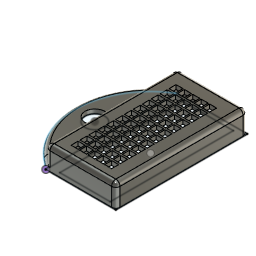
toe-chassis_v1 (Autodesk Fusion 360 design; units mm, degrees)
Autodesk Fusion 360 part; units mm, degrees
sketch "Sketch1" plane through (0, 0, 0) normal (0, 0, 1) x (1, 0, 0)
  line L0 (0, 0) -> (25, 0)
  line L1 (25, 0) -> (25, 47)
  line L2 (25, 47) -> (0, 47)
  line L3 (0, 47) -> (0, 0)
  line L4 (3.5, 1.5) -> (21.5, 1.5)
  line L5 (21.5, 1.5) -> (21.5, 45.5)
  line L6 (21.5, 45.5) -> (3.5, 45.5)
  line L7 (3.5, 45.5) -> (3.5, 1.5)
  line L8 (0, 47) -> (-0.5238, 46.6753)
  line L9 (-3.5824, 2.9853) -> (0, 0)
  arc A0 (-0.5238, 46.6753) -> (-3.5824, 2.9853) centre (13.7026, 23.7273) ccw
  circle A1 centre (-6, 23.5) radius 3.5
  dimension "d1" = 25
  dimension "d2" = 47
  dimension "d3" = 18
  dimension "d4" = 44
  dimension "d5" = 1.5
  dimension "d6" = 3.5
  dimension "d7" = 27
  dimension "d19" = 7
  dimension "d20" = 6
  dimension "d21" = 23.5
  constraint horizontal L0
  constraint vertical L1
  constraint horizontal L2
  constraint vertical L3
  constraint coincident L0.start L3.end
  constraint horizontal L4
  constraint vertical L5
  constraint horizontal L6
  constraint vertical L7
  constraint tangent L9 A0
  constraint tangent L8 A0
  measures "d1" distance of L1.end L2.end
  measures "d2" distance of L0.end L1.end
  measures "d3" distance of L5.end L6.end
  measures "d4" distance of L4.end L5.end
  measures "d5" distance of L2 L6
  measures "d6" distance of L1 L5
  measures "d7" radius of A0
  measures "d19" diameter of A1
  measures "d20" distance of L3 A1.centre
  measures "d21" distance of L2 A1.centre
extrude "Extrude1" add sketch "Sketch1" along normal blind 1.5 contours L0 L1 L2 L3 | L3 L8 L9 A0 | L4 L5 L6 L7 | A1
extrude "Extrude2" add sketch "Sketch1" along normal blind 8 contours L0 L1 L2 L3 | L4 L5 L6 L7
extrude "Extrude3" cut sketch "Sketch1" along normal blind 6.5 contours L4 L5 L6 L7
sketch "Sketch3" plane through (0, 47, 0) normal (0, 1, 0) x (-1, 0, 0)
  line L0 (-25, 0) -> (0, 0)
  line L1 (0, 0) -> (0, 1.5)
  line L2 (0, 1.5) -> (0, 8)
  line L3 (0, 8) -> (-25, 8)
  line L4 (-25, 8) -> (-25, 0)
  line L5 (-17, 0) -> (-8, 0)
  line L6 (-8, 0) -> (-8, 5)
  line L7 (-8, 5) -> (-17, 5)
  line L8 (-17, 5) -> (-17, 0)
  dimension "d14" = 9
  dimension "d15" = 5
  dimension "d16" = 8
  constraint horizontal L5
  constraint vertical L6
  constraint horizontal L7
  constraint vertical L8
  constraint coincident L0 L5.start
  measures "d14" distance of L6.end L7.end
  measures "d15" distance of L5.end L6.end
  measures "d16" distance of L4 L8
extrude "Extrude4" cut sketch "Sketch3" against normal blind 6 contours L0 L5 L6 L7 L8
extrude "Extrude5" cut sketch "Sketch1" along normal blind 8 contours A1
fillet "Fillet1" radius 1.5 8 edges at (0, 47, 4.75) (12.5, 47, 8) (25, 47, 4) (0, 23.5, 8) (25, 23.5, 8) (25, 0, 4) (12.5, 0, 8) (0, 0, 4.75)
fillet "Fillet2" radius 1.5 3 edges at (-0.2619, 46.8376, 1.5) (-13.2315, 25.6129, 1.5) (-1.7912, 1.4927, 1.5)
sketch "Sketch4" plane through (0, 0, 8) normal (0, 0, 1) x (-1, 0, 0)
  line L0 (-1.5, -1.5) -> (-23.5, -1.5)
  line L1 (-23.5, -1.5) -> (-23.5, -45.5)
  line L2 (-23.5, -45.5) -> (-1.5, -45.5)
  line L3 (-1.5, -45.5) -> (-1.5, -1.5)
  line L4 (-19.5, -41.5) -> (-17, -41.5)
  line L5 (-17, -41.5) -> (-17, -39)
  line L6 (-17, -39) -> (-19.5, -39)
  line L7 (-19.5, -39) -> (-19.5, -41.5)
  line L8 (-14, -39) -> (-16.5, -39)
  line L9 (-14, -41.5) -> (-14, -39)
  line L10 (-16.5, -41.5) -> (-14, -41.5)
  line L11 (-16.5, -39) -> (-16.5, -41.5)
  line L12 (-11, -39) -> (-13.5, -39)
  line L13 (-11, -41.5) -> (-11, -39)
  line L14 (-13.5, -41.5) -> (-11, -41.5)
  line L15 (-13.5, -39) -> (-13.5, -41.5)
  line L16 (-8, -39) -> (-10.5, -39)
  line L17 (-8, -41.5) -> (-8, -39)
  line L18 (-10.5, -41.5) -> (-8, -41.5)
  line L19 (-10.5, -39) -> (-10.5, -41.5)
  line L20 (-5, -39) -> (-7.5, -39)
  line L21 (-5, -41.5) -> (-5, -39)
  line L22 (-7.5, -41.5) -> (-5, -41.5)
  line L23 (-7.5, -39) -> (-7.5, -41.5)
  line L24 (-17, -35.8182) -> (-19.5, -35.8182)
  line L25 (-17, -38.3182) -> (-17, -35.8182)
  line L26 (-19.5, -38.3182) -> (-17, -38.3182)
  line L27 (-19.5, -35.8182) -> (-19.5, -38.3182)
  line L28 (-14, -35.8182) -> (-16.5, -35.8182)
  line L29 (-14, -38.3182) -> (-14, -35.8182)
  line L30 (-16.5, -38.3182) -> (-14, -38.3182)
  line L31 (-16.5, -35.8182) -> (-16.5, -38.3182)
  line L32 (-11, -35.8182) -> (-13.5, -35.8182)
  line L33 (-11, -38.3182) -> (-11, -35.8182)
  line L34 (-13.5, -38.3182) -> (-11, -38.3182)
  line L35 (-13.5, -35.8182) -> (-13.5, -38.3182)
  line L36 (-8, -35.8182) -> (-10.5, -35.8182)
  line L37 (-8, -38.3182) -> (-8, -35.8182)
  line L38 (-10.5, -38.3182) -> (-8, -38.3182)
  line L39 (-10.5, -35.8182) -> (-10.5, -38.3182)
  line L40 (-5, -35.8182) -> (-7.5, -35.8182)
  line L41 (-5, -38.3182) -> (-5, -35.8182)
  line L42 (-7.5, -38.3182) -> (-5, -38.3182)
  line L43 (-7.5, -35.8182) -> (-7.5, -38.3182)
  line L44 (-17, -32.6364) -> (-19.5, -32.6364)
  line L45 (-17, -35.1364) -> (-17, -32.6364)
  line L46 (-19.5, -35.1364) -> (-17, -35.1364)
  line L47 (-19.5, -32.6364) -> (-19.5, -35.1364)
  line L48 (-14, -32.6364) -> (-16.5, -32.6364)
  line L49 (-14, -35.1364) -> (-14, -32.6364)
  line L50 (-16.5, -35.1364) -> (-14, -35.1364)
  line L51 (-16.5, -32.6364) -> (-16.5, -35.1364)
  line L52 (-11, -32.6364) -> (-13.5, -32.6364)
  line L53 (-11, -35.1364) -> (-11, -32.6364)
  line L54 (-13.5, -35.1364) -> (-11, -35.1364)
  line L55 (-13.5, -32.6364) -> (-13.5, -35.1364)
  line L56 (-8, -32.6364) -> (-10.5, -32.6364)
  line L57 (-8, -35.1364) -> (-8, -32.6364)
  line L58 (-10.5, -35.1364) -> (-8, -35.1364)
  line L59 (-10.5, -32.6364) -> (-10.5, -35.1364)
  line L60 (-5, -32.6364) -> (-7.5, -32.6364)
  line L61 (-5, -35.1364) -> (-5, -32.6364)
  line L62 (-7.5, -35.1364) -> (-5, -35.1364)
  line L63 (-7.5, -32.6364) -> (-7.5, -35.1364)
  line L64 (-17, -29.4545) -> (-19.5, -29.4545)
  line L65 (-17, -31.9545) -> (-17, -29.4545)
  line L66 (-19.5, -31.9545) -> (-17, -31.9545)
  line L67 (-19.5, -29.4545) -> (-19.5, -31.9545)
  line L68 (-14, -29.4545) -> (-16.5, -29.4545)
  line L69 (-14, -31.9545) -> (-14, -29.4545)
  line L70 (-16.5, -31.9545) -> (-14, -31.9545)
  line L71 (-16.5, -29.4545) -> (-16.5, -31.9545)
  line L72 (-11, -29.4545) -> (-13.5, -29.4545)
  line L73 (-11, -31.9545) -> (-11, -29.4545)
  line L74 (-13.5, -31.9545) -> (-11, -31.9545)
  line L75 (-13.5, -29.4545) -> (-13.5, -31.9545)
  line L76 (-8, -29.4545) -> (-10.5, -29.4545)
  line L77 (-8, -31.9545) -> (-8, -29.4545)
  line L78 (-10.5, -31.9545) -> (-8, -31.9545)
  line L79 (-10.5, -29.4545) -> (-10.5, -31.9545)
  line L80 (-5, -29.4545) -> (-7.5, -29.4545)
  line L81 (-5, -31.9545) -> (-5, -29.4545)
  line L82 (-7.5, -31.9545) -> (-5, -31.9545)
  line L83 (-7.5, -29.4545) -> (-7.5, -31.9545)
  line L84 (-17, -26.2727) -> (-19.5, -26.2727)
  line L85 (-17, -28.7727) -> (-17, -26.2727)
  line L86 (-19.5, -28.7727) -> (-17, -28.7727)
  line L87 (-19.5, -26.2727) -> (-19.5, -28.7727)
  line L88 (-14, -26.2727) -> (-16.5, -26.2727)
  line L89 (-14, -28.7727) -> (-14, -26.2727)
  line L90 (-16.5, -28.7727) -> (-14, -28.7727)
  line L91 (-16.5, -26.2727) -> (-16.5, -28.7727)
  line L92 (-11, -26.2727) -> (-13.5, -26.2727)
  line L93 (-11, -28.7727) -> (-11, -26.2727)
  line L94 (-13.5, -28.7727) -> (-11, -28.7727)
  line L95 (-13.5, -26.2727) -> (-13.5, -28.7727)
  line L96 (-8, -26.2727) -> (-10.5, -26.2727)
  line L97 (-8, -28.7727) -> (-8, -26.2727)
  line L98 (-10.5, -28.7727) -> (-8, -28.7727)
  line L99 (-10.5, -26.2727) -> (-10.5, -28.7727)
  line L100 (-5, -26.2727) -> (-7.5, -26.2727)
  line L101 (-5, -28.7727) -> (-5, -26.2727)
  line L102 (-7.5, -28.7727) -> (-5, -28.7727)
  line L103 (-7.5, -26.2727) -> (-7.5, -28.7727)
  line L104 (-17, -23.0909) -> (-19.5, -23.0909)
  line L105 (-17, -25.5909) -> (-17, -23.0909)
  line L106 (-19.5, -25.5909) -> (-17, -25.5909)
  line L107 (-19.5, -23.0909) -> (-19.5, -25.5909)
  line L108 (-14, -23.0909) -> (-16.5, -23.0909)
  line L109 (-14, -25.5909) -> (-14, -23.0909)
  line L110 (-16.5, -25.5909) -> (-14, -25.5909)
  line L111 (-16.5, -23.0909) -> (-16.5, -25.5909)
  line L112 (-11, -23.0909) -> (-13.5, -23.0909)
  line L113 (-11, -25.5909) -> (-11, -23.0909)
  line L114 (-13.5, -25.5909) -> (-11, -25.5909)
  line L115 (-13.5, -23.0909) -> (-13.5, -25.5909)
  line L116 (-8, -23.0909) -> (-10.5, -23.0909)
  line L117 (-8, -25.5909) -> (-8, -23.0909)
  line L118 (-10.5, -25.5909) -> (-8, -25.5909)
  line L119 (-10.5, -23.0909) -> (-10.5, -25.5909)
  line L120 (-5, -23.0909) -> (-7.5, -23.0909)
  line L121 (-5, -25.5909) -> (-5, -23.0909)
  line L122 (-7.5, -25.5909) -> (-5, -25.5909)
  line L123 (-7.5, -23.0909) -> (-7.5, -25.5909)
  line L124 (-17, -19.9091) -> (-19.5, -19.9091)
  line L125 (-17, -22.4091) -> (-17, -19.9091)
  line L126 (-19.5, -22.4091) -> (-17, -22.4091)
  line L127 (-19.5, -19.9091) -> (-19.5, -22.4091)
  line L128 (-14, -19.9091) -> (-16.5, -19.9091)
  line L129 (-14, -22.4091) -> (-14, -19.9091)
  line L130 (-16.5, -22.4091) -> (-14, -22.4091)
  line L131 (-16.5, -19.9091) -> (-16.5, -22.4091)
  line L132 (-11, -19.9091) -> (-13.5, -19.9091)
  line L133 (-11, -22.4091) -> (-11, -19.9091)
  line L134 (-13.5, -22.4091) -> (-11, -22.4091)
  line L135 (-13.5, -19.9091) -> (-13.5, -22.4091)
  line L136 (-8, -19.9091) -> (-10.5, -19.9091)
  line L137 (-8, -22.4091) -> (-8, -19.9091)
  line L138 (-10.5, -22.4091) -> (-8, -22.4091)
  line L139 (-10.5, -19.9091) -> (-10.5, -22.4091)
  line L140 (-5, -19.9091) -> (-7.5, -19.9091)
  line L141 (-5, -22.4091) -> (-5, -19.9091)
  line L142 (-7.5, -22.4091) -> (-5, -22.4091)
  line L143 (-7.5, -19.9091) -> (-7.5, -22.4091)
  line L144 (-17, -16.7273) -> (-19.5, -16.7273)
  line L145 (-17, -19.2273) -> (-17, -16.7273)
  line L146 (-19.5, -19.2273) -> (-17, -19.2273)
  line L147 (-19.5, -16.7273) -> (-19.5, -19.2273)
  line L148 (-14, -16.7273) -> (-16.5, -16.7273)
  line L149 (-14, -19.2273) -> (-14, -16.7273)
  line L150 (-16.5, -19.2273) -> (-14, -19.2273)
  line L151 (-16.5, -16.7273) -> (-16.5, -19.2273)
  line L152 (-11, -16.7273) -> (-13.5, -16.7273)
  line L153 (-11, -19.2273) -> (-11, -16.7273)
  line L154 (-13.5, -19.2273) -> (-11, -19.2273)
  line L155 (-13.5, -16.7273) -> (-13.5, -19.2273)
  line L156 (-8, -16.7273) -> (-10.5, -16.7273)
  line L157 (-8, -19.2273) -> (-8, -16.7273)
  line L158 (-10.5, -19.2273) -> (-8, -19.2273)
  line L159 (-10.5, -16.7273) -> (-10.5, -19.2273)
  line L160 (-5, -16.7273) -> (-7.5, -16.7273)
  line L161 (-5, -19.2273) -> (-5, -16.7273)
  line L162 (-7.5, -19.2273) -> (-5, -19.2273)
  line L163 (-7.5, -16.7273) -> (-7.5, -19.2273)
  line L164 (-17, -13.5455) -> (-19.5, -13.5455)
  line L165 (-17, -16.0455) -> (-17, -13.5455)
  line L166 (-19.5, -16.0455) -> (-17, -16.0455)
  line L167 (-19.5, -13.5455) -> (-19.5, -16.0455)
  line L168 (-14, -13.5455) -> (-16.5, -13.5455)
  line L169 (-14, -16.0455) -> (-14, -13.5455)
  line L170 (-16.5, -16.0455) -> (-14, -16.0455)
  line L171 (-16.5, -13.5455) -> (-16.5, -16.0455)
  line L172 (-11, -13.5455) -> (-13.5, -13.5455)
  line L173 (-11, -16.0455) -> (-11, -13.5455)
  line L174 (-13.5, -16.0455) -> (-11, -16.0455)
  line L175 (-13.5, -13.5455) -> (-13.5, -16.0455)
  line L176 (-8, -13.5455) -> (-10.5, -13.5455)
  line L177 (-8, -16.0455) -> (-8, -13.5455)
  line L178 (-10.5, -16.0455) -> (-8, -16.0455)
  line L179 (-10.5, -13.5455) -> (-10.5, -16.0455)
  line L180 (-5, -13.5455) -> (-7.5, -13.5455)
  line L181 (-5, -16.0455) -> (-5, -13.5455)
  line L182 (-7.5, -16.0455) -> (-5, -16.0455)
  line L183 (-7.5, -13.5455) -> (-7.5, -16.0455)
  line L184 (-17, -10.3636) -> (-19.5, -10.3636)
  line L185 (-17, -12.8636) -> (-17, -10.3636)
  line L186 (-19.5, -12.8636) -> (-17, -12.8636)
  line L187 (-19.5, -10.3636) -> (-19.5, -12.8636)
  line L188 (-14, -10.3636) -> (-16.5, -10.3636)
  line L189 (-14, -12.8636) -> (-14, -10.3636)
  line L190 (-16.5, -12.8636) -> (-14, -12.8636)
  line L191 (-16.5, -10.3636) -> (-16.5, -12.8636)
  line L192 (-11, -10.3636) -> (-13.5, -10.3636)
  line L193 (-11, -12.8636) -> (-11, -10.3636)
  line L194 (-13.5, -12.8636) -> (-11, -12.8636)
  line L195 (-13.5, -10.3636) -> (-13.5, -12.8636)
  line L196 (-8, -10.3636) -> (-10.5, -10.3636)
  line L197 (-8, -12.8636) -> (-8, -10.3636)
  line L198 (-10.5, -12.8636) -> (-8, -12.8636)
  line L199 (-10.5, -10.3636) -> (-10.5, -12.8636)
  line L200 (-5, -10.3636) -> (-7.5, -10.3636)
  line L201 (-5, -12.8636) -> (-5, -10.3636)
  line L202 (-7.5, -12.8636) -> (-5, -12.8636)
  line L203 (-7.5, -10.3636) -> (-7.5, -12.8636)
  line L204 (-17, -7.1818) -> (-19.5, -7.1818)
  line L205 (-17, -9.6818) -> (-17, -7.1818)
  line L206 (-19.5, -9.6818) -> (-17, -9.6818)
  line L207 (-19.5, -7.1818) -> (-19.5, -9.6818)
  line L208 (-14, -7.1818) -> (-16.5, -7.1818)
  line L209 (-14, -9.6818) -> (-14, -7.1818)
  line L210 (-16.5, -9.6818) -> (-14, -9.6818)
  line L211 (-16.5, -7.1818) -> (-16.5, -9.6818)
  line L212 (-11, -7.1818) -> (-13.5, -7.1818)
  line L213 (-11, -9.6818) -> (-11, -7.1818)
  line L214 (-13.5, -9.6818) -> (-11, -9.6818)
  line L215 (-13.5, -7.1818) -> (-13.5, -9.6818)
  line L216 (-8, -7.1818) -> (-10.5, -7.1818)
  line L217 (-8, -9.6818) -> (-8, -7.1818)
  line L218 (-10.5, -9.6818) -> (-8, -9.6818)
  line L219 (-10.5, -7.1818) -> (-10.5, -9.6818)
  line L220 (-5, -7.1818) -> (-7.5, -7.1818)
  line L221 (-5, -9.6818) -> (-5, -7.1818)
  line L222 (-7.5, -9.6818) -> (-5, -9.6818)
  line L223 (-7.5, -7.1818) -> (-7.5, -9.6818)
  line L224 (-17, -4) -> (-19.5, -4)
  line L225 (-17, -6.5) -> (-17, -4)
  line L226 (-19.5, -6.5) -> (-17, -6.5)
  line L227 (-19.5, -4) -> (-19.5, -6.5)
  line L228 (-14, -4) -> (-16.5, -4)
  line L229 (-14, -6.5) -> (-14, -4)
  line L230 (-16.5, -6.5) -> (-14, -6.5)
  line L231 (-16.5, -4) -> (-16.5, -6.5)
  line L232 (-11, -4) -> (-13.5, -4)
  line L233 (-11, -6.5) -> (-11, -4)
  line L234 (-13.5, -6.5) -> (-11, -6.5)
  line L235 (-13.5, -4) -> (-13.5, -6.5)
  line L236 (-8, -4) -> (-10.5, -4)
  line L237 (-8, -6.5) -> (-8, -4)
  line L238 (-10.5, -6.5) -> (-8, -6.5)
  line L239 (-10.5, -4) -> (-10.5, -6.5)
  line L240 (-5, -4) -> (-7.5, -4)
  line L241 (-5, -6.5) -> (-5, -4)
  line L242 (-7.5, -6.5) -> (-5, -6.5)
  line L243 (-7.5, -4) -> (-7.5, -6.5)
  dimension "d28" = 2.5
  dimension "d29" = 2.5
  dimension "d30" = 4
  dimension "d31" = 4
  dimension "d34" = 12
  dimension "d35" = 35
  constraint horizontal L4
  constraint vertical L5
  constraint horizontal L6
  constraint vertical L7
  measures "d28" distance of L4.start L6.end
  measures "d29" distance of L4.start L4.end
  measures "d30" distance of L2 L4
  measures "d31" distance of L1 L7
extrude "Extrude6" cut sketch "Sketch4" against normal blind 30 contours L4 L5 L6 L7 | L8 L9 L10 L11 | L12 L13 L14 L15 | L16 L17 L18 L19 | L20 L21 L22 L23 | L24 L25 L26 L27 | L28 L29 L30 L31 | L32 L33 L34 L35 | L36 L37 L38 L39 | L40 L41 L42 L43 | L44 L45 L46 L47 | L48 L49 L50 L51 | L52 L53 L54 L55 | L56 L57 L58 L59 | L60 L61 L62 L63 | L64 L65 L66 L67 | L68 L69 L70 L71 | L72 L73 L74 L75 | L76 L77 L78 L79 | L80 L81 L82 L83 | L84 L85 L86 L87 | L88 L89 L90 L91 | L92 L93 L94 L95 | L96 L97 L98 L99 | L100 L101 L102 L103 | L104 L105 L106 L107 | L108 L109 L110 L111 | L112 L113 L114 L115 | L116 L117 L118 L119 | L120 L121 L122 L123 | L124 L125 L126 L127 | L128 L129 L130 L131 | L132 L133 L134 L135 | L136 L137 L138 L139 | L140 L141 L142 L143 | L144 L145 L146 L147 | L148 L149 L150 L151 | L152 L153 L154 L155 | L156 L157 L158 L159 | L160 L161 L162 L163 | L164 L165 L166 L167 | L168 L169 L170 L171 | L172 L173 L174 L175 | L176 L177 L178 L179 | L180 L181 L182 L183 | L184 L185 L186 L187 | L188 L189 L190 L191 | L192 L193 L194 L195 | L196 L197 L198 L199 | L200 L201 L202 L203 | L204 L205 L206 L207 | L208 L209 L210 L211 | L212 L213 L214 L215 | L216 L217 L218 L219 | L220 L221 L222 L223 | L224 L225 L226 L227 | L228 L229 L230 L231 | L232 L233 L234 L235 | L236 L237 L238 L239 | L240 L241 L242 L243
